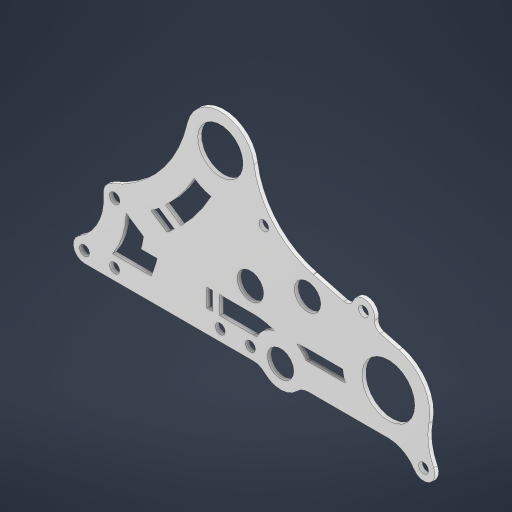
# Autodesk Inventor part: reservoir_mount
Saved by Autodesk Inventor 2024 (Build 280153000, 153)
## iProperties
Created: 2023-11-18
Part Number: reservoir_mount
Material: Acetal Resin, White
Document SubType Name: Sheet Metal
Designer: avere
Density: 1.425 g/cm^3
Appearance: Smooth - White
Flat Pattern Width: 9.19608 cm
Flat Pattern Length: 15.2289 cm
Flat Pattern Area: 140.046 cm^2
Sheet Metal Rule: Default_mm
Sheet Metal Width: 3.621 in
Sheet Metal Length: 5.996 in
Sheet Metal Area: 21.707 in^2
Author: avere
Autodesk Inventor part; units mm, degrees
ref_plane "YZ Plane" through (0, 0, 0) normal (1, 0, 0) x (0, 1, 0)
ref_plane "XZ Plane" through (0, 0, 0) normal (0, 1, 0) x (-1, 0, 0)
ref_plane "XY Plane" through (0, 0, 0) normal (0, 0, 1) x (1, 0, 0)
sketch "main" plane through (0, 0, 0) normal (0, 0, 1) x (1, 0, 0)
  circle A0 centre (-14.2783, -9.7185) radius 2.1844
  ellipse E0 centre (34.925, 23.8125) end of major axis (34.925, 33.3375) minor radius 9.5235
  point P0 (-4.2471, 2.7063)
sketch "Sketch1" plane through (0, 0, 0) normal (0, 0, 1) x (1, 0, 0)
  arc A0 (-1.8077, 4.4061) -> (-4.7431, -0.4299) centre (0, 0) ccw
  arc A1 (58.6308, 41.6064) -> (30.55, 42.7109) centre (44.4887, 39.5733) ccw
  circle A2 centre (0, -25.4) radius 2.0955
  circle A3 centre (-12.7, -25.4) radius 2.0955
  arc A4 (-15.2019, -21.3476) -> (-12.7, -30.1625) centre (-12.7, -25.4) ccw
  line L0 (-12.7, -30.1625) -> (-11.7807, -30.1625)
  arc A5 (-15.2019, -21.3476) -> (-4.7431, -0.4299) centre (-26.8773, -2.4363) ccw
  arc A6 (-1.8077, 4.4061) -> (30.55, 42.7109) centre (-22.4149, 54.6332) ccw
  line L1 (31.75, -25.4) -> (57.15, -25.4) construction
  line L2 (31.75, -25.4) -> (36.5125, -25.4) construction
  circle A7 centre (44.45, -25.4) radius 2.0955
  circle A8 centre (57.15, -25.4) radius 2.0955
  circle A9 centre (69.85, -25.4) radius 5.5499
  arc A10 (63.0478, -32.0675) -> (76.8244, -31.8872) centre (69.85, -25.4) ccw
  circle A11 centre (57.15, -3.403) radius 5.5499
  line L3 (-11.7807, -30.1625) -> (58.513, -30.1625)
  line L4 (81.474, -29.8619) -> (115.2189, -29.8619)
  line L5 (-11.7807, -30.1625) -> (61.6011, -30.1625) construction
  line L6 (78.2653, -29.8619) -> (115.2189, -29.8619) construction
  circle A12 centre (81.2023, 4.7609) radius 5.5499
  arc A13 (83.6265, 13.9723) -> (83.523, 13.9989) centre (81.2023, 4.7609) ccw
  arc A14 (58.6308, 41.6064) -> (83.523, 13.9989) centre (91.6512, 46.3534) ccw
  arc A15 (81.474, -29.8619) -> (76.8244, -31.8872) centre (81.474, -36.2119) ccw
  arc A16 (63.0478, -32.0675) -> (58.513, -30.1625) centre (58.513, -36.5125) ccw
  circle A17 centre (115.2189, -12.3994) radius 11.0998
  arc A18 (132.3184, -15.9417) -> (119.6634, 4.488) centre (115.2189, -12.3994) ccw
  circle A19 centre (104.775, 11.1125) radius 2.0955
  arc A20 (109.4545, 10.2271) -> (100.2659, 12.6454) centre (104.775, 11.1125) ccw
  line L7 (119.6634, 4.488) -> (111.766, 6.5664)
  line L8 (96.4518, 10.5969) -> (83.6265, 13.9723)
  arc A21 (96.4518, 10.5969) -> (100.2659, 12.6454) centre (97.2599, 13.6673) ccw
  arc A22 (109.4545, 10.2271) -> (111.766, 6.5664) centre (112.5741, 9.6369) ccw
  circle A23 centre (130.0641, -33.3375) radius 2.0955
  arc A24 (126.0228, -35.8574) -> (134.3205, -31.2011) centre (130.0641, -33.3375) ccw
  arc A25 (132.3184, -15.9417) -> (134.3205, -31.2011) centre (155.2553, -20.6933) ccw
  arc A26 (126.0228, -35.8574) -> (115.2189, -29.8619) centre (115.2189, -42.5941) ccw
  arc A27 (122.2659, -20.9753) -> (122.2726, -21.4129) centre (155.2553, -20.6933) ccw
  arc A28 (59.7857, -20.6886) -> (58.513, -20.6375) centre (58.513, -36.5125) ccw
  arc A29 (-0.8623, -20.6375) -> (4.8666, -3.0564) centre (-26.8773, -2.4363) ccw
  arc A30 (67.0849, -14.637) -> (58.513, -13.0175) centre (58.513, -36.5125) ccw
  arc A31 (11.0441, -13.0175) -> (12.1111, -7.9042) centre (-26.8773, -2.4363) ccw
  line L9 (4.8666, -3.0564) -> (12.1111, -7.9042)
  line L10 (18.5803, 5.7275) -> (25.1468, 1.3334)
  line L11 (21.4396, 8.2742) -> (27.9161, 3.9403)
  arc A32 (15.3458, -20.6375) -> (17.8676, -13.0175) centre (-26.8773, -2.4363) ccw
  line L12 (17.8676, -13.0175) -> (11.0441, -13.0175)
  line L13 (15.3458, -20.6375) -> (-0.8623, -20.6375)
  line L14 (38.7856, -20.6375) -> (38.7856, -13.0175)
  line L15 (41.1925, -20.6375) -> (41.1925, -13.0175)
  line L16 (44.2415, -13.0175) -> (44.2415, -20.6375)
  line L17 (58.513, -13.0175) -> (44.2415, -13.0175)
  line L18 (41.1925, -13.0175) -> (38.7856, -13.0175)
  line L19 (58.513, -20.6375) -> (44.2415, -20.6375)
  line L20 (41.1925, -20.6375) -> (38.7856, -20.6375)
  arc A33 (41.2533, 43.0681) -> (41.1925, 43.0108) centre (44.4887, 39.5733) ccw
  line L21 (15.3458, 3.189) -> (22.0356, -1.2876)
  arc A34 (15.3458, 3.189) -> (18.5803, 5.7275) centre (-22.4149, 54.6332) ccw
  arc A35 (21.4396, 8.2742) -> (33.5532, 23.9747) centre (-22.4149, 54.6332) ccw
  arc A36 (22.0356, -1.2876) -> (25.1468, 1.3334) centre (-22.4149, 54.6332) ccw
  arc A37 (40.5702, 20.9307) -> (41.1925, 20.8107) centre (44.4887, 39.5733) ccw
  arc A38 (27.9161, 3.9403) -> (40.5702, 20.9307) centre (-22.4149, 54.6332) ccw
  arc A39 (33.5532, 23.9747) -> (40.5702, 20.9307) centre (44.4887, 39.5733) ccw
  arc A40 (83.6265, 13.9723) -> (83.523, 13.9989) centre (81.2023, 4.7609) ccw
  arc A41 (67.0849, -14.637) -> (59.7857, -20.6886) centre (69.85, -25.4) ccw
  arc A42 (59.8098, -30.1625) -> (59.882, -30.3118) centre (69.85, -25.4) ccw
  arc A43 (79.9432, -30.0492) -> (80.0274, -29.8619) centre (69.85, -25.4) ccw
  arc A44 (81.474, -14.2875) -> (76.801, -14.7913) centre (81.474, -36.2119) ccw
  arc A45 (80.6713, -18.7848) -> (76.801, -14.7913) centre (69.85, -25.4) ccw
  arc A46 (81.474, -18.7664) -> (80.6713, -18.7848) centre (81.474, -36.2119) ccw
  line L22 (81.474, -18.7664) -> (97.0069, -18.7664)
  arc A47 (96.0187, -14.2875) -> (97.0069, -18.7664) centre (115.2189, -12.3994) ccw
  line L23 (96.0187, -14.2875) -> (81.474, -14.2875)
  circle A48 centre (62.7575, 21.436) radius 2.0955
  circle A49 centre (0, 0) radius 2.1844
  ellipse E0 centre (44.4887, 39.5733) end of major axis (43.2652, 49.0194) minor radius 9.5235
  point P0 (107.9569, 7.5689)
  point P1 (100.2609, 9.5944)
  dimension "d1" = 9.525
  dimension "d2" = 28.575
  dimension "d7" = 22.225
  dimension "d25" = 4.191
  dimension "d26" = 4.191
  dimension "d30" = 11.0998
  dimension "d31" = 11.0998
  dimension "d38" = 6.35
  dimension "d43" = 4.191
  dimension "d44" = 9.525
  dimension "d47" = 9.525
  dimension "d54" = 4.191
  constraints: 82 point on circle, 48 centre point, 48 end point, 23 tangent, 13 horizontal, 10 coincident, 8 point on line, 6 perpendicular, 3 parallel, 2 equal radius, 1 concentric, 1 midpoint, 12 other
  measures "d1" diameter of A0
  measures "d2" diameter of A1
  measures "d7" radius of A5
  measures "d25" diameter of A7
  measures "d26" diameter of A8
  measures "d30" diameter of A9
  measures "d31" diameter of A11
  measures "d38" radius of A15
  measures "d43" diameter of A19
  measures "d44" diameter of A20
  measures "d47" diameter of A24
  measures "d54" diameter of A48
extrude "Extrusion1" add sketch "Sketch1" along normal blind 1.5875
body "Solid1"
